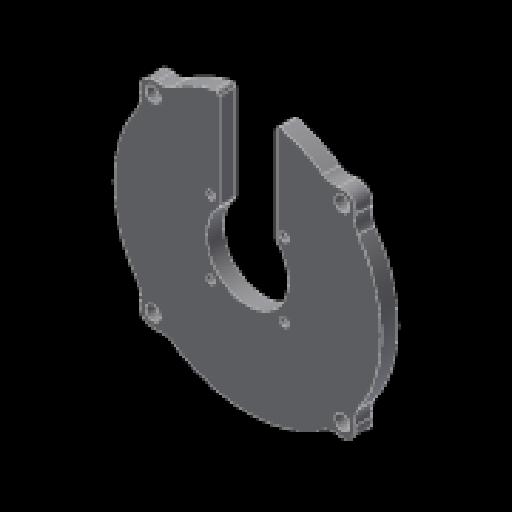
# Autodesk Inventor part: CimCoderMount
Saved by Autodesk Inventor 2025.2 (Build 292293000, 293)
## iProperties
Created: 2026-01-26
Part Number: CimCoderMount
Material: Generic
Document SubType Name: Sheet Metal
Designer: valer
Density: 1 g/cm^3
Appearance: Default
Sheet Metal Rule: Default
Author: valer
Autodesk Inventor part; units mm, degrees
ref_plane "YZ Plane" through (0, 0, 0) normal (1, 0, 0) x (0, 1, 0)
ref_plane "XZ Plane" through (0, 0, 0) normal (0, 1, 0) x (-1, 0, 0)
ref_plane "XY Plane" through (0, 0, 0) normal (0, 0, 1) x (1, 0, 0)
sketch "Base" plane through (0, 0, 0) normal (0, 0, 1) x (1, 0, 0)
  circle A0 centre (0, 0) radius 50.8
  circle A1 centre (0, 0) radius 16.5 construction
  line L0 (-71.12, 0) -> (71.12, 0)
  line L1 (0, -71.12) -> (0, 71.12) construction
  circle A2 centre (0, 0) radius 16 construction
  circle A3 centre (0, 0) radius 40
  line L2 (0, 0) -> (28.2843, 28.2843) construction
  circle A4 centre (28.2843, 28.2843) radius 2.2
  circle A5 centre (-28.2843, 28.2843) radius 2.2
  circle A6 centre (28.2843, -28.2843) radius 2.2
  circle A7 centre (-28.2843, -28.2843) radius 2.2
  circle A8 centre (28.2843, 28.2843) radius 4
  circle A9 centre (-28.2843, 28.2843) radius 4
  line L3 (0, 0) -> (35.921, 35.921)
  line L4 (0, 0) -> (-35.921, 35.921) construction
  circle A10 centre (28.2843, -28.2843) radius 4
  circle A11 centre (-28.2843, -28.2843) radius 4
  circle A12 centre (0, 0) radius 18.5
  circle A13 centre (-10.975, -11) radius 1.25
  circle A14 centre (10.975, -11) radius 1.25
  circle A15 centre (10.975, 11) radius 1.25
  circle A16 centre (-10.975, 11) radius 1.25
  circle A17 centre (0, 0) radius 12.2174
  point P0 (-25.4558, 25.4558)
  point P1 (-11.6673, 11.6673)
  point P2 (11.6673, 11.6673)
  point P3 (25.4558, 25.4558)
  point P4 (31.1127, 31.1127)
  point P5 (-31.1127, 31.1127)
  point P6 (25.318, 30.9677)
  point P7 (-25.318, 30.9677)
  point P8 (-30.9677, 25.318)
  point P9 (-40, 0)
  point P10 (-16.5, 0)
  point P11 (16.5, 0)
  point P12 (40, 0)
  point P13 (30.9677, 25.318)
  point P14 (30.9677, -25.318)
  point P15 (-30.9677, -25.318)
  point P16 (-25.318, -30.9677)
  point P17 (25.318, -30.9677)
  point P18 (-29.7965, 26.6864)
  point P19 (-26.6864, 29.7965)
  point P20 (-26.6864, -29.7965)
  point P21 (-29.7965, -26.6864)
extrude "Plate1" add sketch "Base" along normal blind 5 contours A3 A10 A11 L0 A12 | L0 A12 L3 A8 A3 | L3 A4 A3 A8 | A8 A3 A4 L3 | A3 A9 A8 L3 A12 L0 | A12 L0 A17 | L0 A17 L3 A15 A12 | A8 L3 A4 A3 | A10 A3 A6 | A3 A6 A10 | A3 A4 L3 A8 | A12 L3 A15 A17 L0 | A9 A3 A5 | A3 A5 A9 | A11 A3 A7 | A3 A7 A11
fillet "FilletsFeature" radius 6 8 edges at (-30.9677, 25.318, 2.5) (-30.9677, -25.318, 2.5) (-25.318, -30.9677, 2.5) (25.318, -30.9677, 2.5) (30.9677, -25.318, 2.5) (30.9677, 25.318, 2.5) (25.318, 30.9677, 2.5) (-25.318, 30.9677, 2.5)
sketch "ConnectorCut" plane through (0, 0, 5) normal (0, 0, 1) x (1, 0, 0)
  line L0 (-8, 0) -> (8, 0)
  line L1 (8, 0) -> (8, 40)
  line L2 (8, 40) -> (-8, 40)
  line L3 (-8, 40) -> (-8, 0)
  line L4 (-7.7989, 12.523) -> (-7.7989, 19.523) projected
  line L5 (7.6211, 12.523) -> (7.6211, 19.523) projected
  arc A0 (-33.0444, 22.5403) -> (-33.0444, -22.5403) centre (0, 0) ccw projected
  point P0 (0, 0)
  point P1 (0, 0)
  point P2 (-22.5403, 33.0444)
  point P3 (22.5403, 33.0444)
  point P4 (8, 39.1918)
  point P5 (-8, 39.1918)
  point P6 (-30.9677, -25.318)
  dimension "d37" = 16
  constraints: 8 end point, 2 parallel, 1 coincident, 1 horizontal, 1 midpoint, 1 perpendicular, 1 tangent
  measures "d37" distance between parallel lines of L1 L3
extrude "ConnectorCutFeature" cut sketch "ConnectorCut" against normal blind 5
fillet "CutFilletsFeature" radius 1 4 edges at (-8, 39.1918, 2.5) (8, 39.1918, 2.5) (-8, 9.2339, 2.5) (8, 9.2339, 2.5)
equation "\"d34\" = Thickness"
equation "\"d28\" = Thickness"
equation "\"BendRadius\" = Thickness"
equation "\"BendReliefWidth\" = Thickness"
equation "\"BendReliefDepth\" = 0.5 * Thickness"
equation "\"TransitionRadius\" = BendRadius"
equation "\"JacobiRadiusSize\" = BendRadius"
equation "\"GapSize\" = Thickness"
equation "\"Thickness\" = 5"
body "Solid2"
